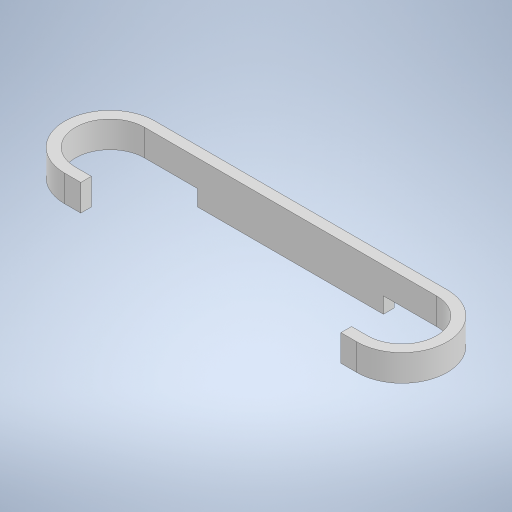
# Autodesk Inventor part: Stand Brace
Saved by Autodesk Inventor 2024.1 (Build 281209000, 209)
## iProperties
Created: 2024-01-03
Part Number: Stand Brace
Material: Generic
Document SubType Name: Modeling
Designer: ryanm
Density: 1 g/cm^3
Appearance: Default
Author: ryanm
Autodesk Inventor part; units mm, degrees
ref_plane "YZ Plane" through (0, 0, 0) normal (1, 0, 0) x (0, 1, 0)
ref_plane "XZ Plane" through (0, 0, 0) normal (0, 1, 0) x (-1, 0, 0)
ref_plane "XY Plane" through (0, 0, 0) normal (0, 0, 1) x (1, 0, 0)
sketch "Sketch1" plane through (0, 0, 0) normal (0, 1, 0) x (-1, 0, 0)
  arc A0 (27.5, -6.5) -> (27.5, 6.5) centre (27.5, 0) ccw
  arc A1 (-27.5, 6.5) -> (-27.5, -6.5) centre (-27.5, 0) ccw
  line L0 (27.5, -6.5) -> (-27.5, -6.5)
  arc A2 (27.5, -8.5) -> (27.5, 8.5) centre (27.5, 0) ccw
  line L1 (27.5, -8.5) -> (-27.5, -8.5)
  arc A3 (-27.5, 8.5) -> (-27.5, -8.5) centre (-27.5, 0) ccw
  line L2 (27.5, 6.5) -> (24.5, 6.5)
  line L3 (24.5, 6.5) -> (24.5, 8.5)
  line L4 (24.5, 8.5) -> (27.5, 8.5)
  line L5 (-27.5, 8.5) -> (-24.5, 8.5)
  line L6 (-24.5, 8.5) -> (-24.5, 6.5)
  line L7 (-24.5, 6.5) -> (-27.5, 6.5)
  point P0 (0, 0)
  point P1 (0, -6.5)
  dimension "d0" = 13
  dimension "d1" = 13
  dimension "d2" = 55
  dimension "d3" = 2
  dimension "d4" = 2
  dimension "d5" = 2
  dimension "d8" = 3
  dimension "d9" = 2
  dimension "d10" = 2
  dimension "d11" = 3
  dimension "d12" = 2
  dimension "d13" = 2
  constraints: 16 end point, 8 point on circle, 4 centre point, 4 perpendicular, 3 horizontal alignment, 2 horizontal, 1 midpoint, 1 parallel, 1 tangent, 1 vertical alignment
  measures "d0" diameter of A0
  measures "d1" diameter of A1
  measures "d2" distance of L0.start L0.end
  measures "d3" radial gap between concentric circles of A0 A2
  measures "d4" distance between parallel lines of L0 L1
  measures "d5" radial gap between concentric circles of A1 A3
  measures "d8" distance of L2.start L2.end
  measures "d9" distance of L2.end L3.end
  measures "d10" distance of L4.end L2.start
  measures "d11" distance of L5.start L5.end
  measures "d12" distance of L5.end L6.end
  measures "d13" distance of L5.start L7.end
extrude "Extrusion1" add sketch "Sketch1" along normal blind 5
sketch "Sketch2" plane through (0, 0, 0) normal (0, -1, 0) x (1, 0, 0)
  line L0 (27.5, -8.5) -> (-27.5, -8.5) projected
  arc A0 (27.5, -8.5) -> (27.5, 8.5) centre (27.5, 0) ccw projected
  line L1 (24.5, 8.5) -> (27.5, 8.5) projected
  line L2 (24.5, 6.5) -> (24.5, 8.5) projected
  line L3 (27.5, 6.5) -> (24.5, 6.5) projected
  arc A1 (27.5, -6.5) -> (27.5, 6.5) centre (27.5, 0) ccw projected
  line L4 (-27.5, -6.5) -> (27.5, -6.5) projected
  arc A2 (-27.5, 6.5) -> (-27.5, -6.5) centre (-27.5, 0) ccw projected
  line L5 (-24.5, 6.5) -> (-27.5, 6.5) projected
  line L6 (-24.5, 8.5) -> (-24.5, 6.5) projected
  line L7 (-27.5, 8.5) -> (-24.5, 8.5) projected
  arc A3 (-27.5, 8.5) -> (-27.5, -8.5) centre (-27.5, 0) ccw projected
  line L8 (-17.5, -6.5) -> (-17.5, -8.5)
  line L9 (17.5, -6.5) -> (17.5, -8.5)
  point P0 (0, 0)
  dimension "d16" = 35
  dimension "d17" = 10
  constraints: 4 end point, 4 point on line, 2 perpendicular
  measures "d16" distance between parallel lines of L9 L8
  measures "d17" distance from line of L8 L0.end
extrude "Extrusion2" add sketch "Sketch2" along normal blind 3 contours L0 L8 L4 L9
equation "\"d1\" = d0"
body "Solid1"
